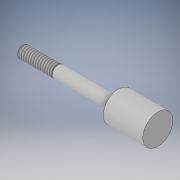
# Autodesk Inventor part: 0070.0110000_rod
Saved by Autodesk Inventor 2018 (Build 220112000, 112)
## iProperties
Created: 2019-01-16
Part Number: 0070.0110000_rod
Material: Generic
Catalog Web Link: www.cadenas.de
Description: Standard Air Cylinder_rod-Original Line - Standard Air Cylinders
Vendor: BIMBA
Document SubType Name: Modeling
Designer: s-4008082
Manufacturer: BIMBA
Mass: 0.744089 g
Surface Area: 6.29772 cm^2
Volume: 0.744089 cm^3
Density: 1 g/cm^3
Appearance: PSOLRGB-181-181-181
Category: PARTsolutions
Company: BIMBA
Title: 0070.0110000_rod
Author: Cadenas PARTsolutions
Comments: Original Line - Standard Air Cylinders
PSOL_IDENT_0: {$CADENAS_DATA\23d-libs\bimba\bimba\bimba_imperial\bimba_full_line\original_line_cylinders\standard_
PSOL_IDENT_1: air_cylinders\rod.prj},325 {VTYP=3D},{NB=0070.0110000_rod},{LINA=0070.0110000_rod},{NN=Standard Air
PSOL_IDENT_2: Cylinder_rod},{DATE=21.03.2018 14:31:21},{GEOMDATE=09.11.2017 13:09:15},{VERSION=},{LINEID=20},{WBVA
PSOL_IDENT_3: R=STROKE,ACTING,MNT,DER,NR,BM,CO,M,EE,EEL,K,Q,Y,F,G,T,B,H,SER,SR,NT,W,E,HL,ST,STP,PRC,PB,COLOR1,FCD,
PSOL_IDENT_4: RCD,BCD},{WBNUMERIC=STROKE,EEL,COLOR1,FCD,RCD,BCD}  {NB=0070.0110000_rod},{LINA=0070.0110000_rod},{K
PSOL_IDENT_5: T=DUMMY},{PN=0070.011000},{DASH=},{BORE=0.31250000},{BOREPN=007},{STROKE=0.011},{STROKEALG=[0.001:50
PSOL_IDENT_6: /0.001]},{STROKE1=0.011},{ACTING=},{ACTINGALG= '' , 'Single Acting' , 'R' , 'Reverse Single Acting'
PSOL_IDENT_7: , 'D' , 'Double Acting' },{ACTINGPN=},{MNT=},{MNTALG= '' , 'Front Nose Mounting' , 'XP' , 'Double En
PSOL_IDENT_8: d or Rear Pivot Mounting' },{TYPE=},{MNTPN=},{DER=},{DERALG= '' , 'N/A' },{NR=},{NRALG= '' , 'N/A' }
PSOL_IDENT_9: ,{NRPN=},{BM=},{BMALG= '' , 'N/A' },{BMPN=},{CO=},{COALG= '' , 'N/A' },{M=},{MALG= '', 'Without Magn
PSOL_IDENT_10: et', 'M', 'With Magnet' },{EE=},{EEL=0},{EEMAX=50},{EEALG= '', 'Without Extra Extension', 'EE', 'Wit
PSOL_IDENT_11: h Extra Extension' },{EELALG=0},{EEPN=},{EEPN1=0.000},{K=},{KALG= '' , 'N/A' },{KPN=},{Q=},{QALG= ''
PSOL_IDENT_12: , 'Without Side Ported Rear Head' , 'Q' , 'With Side Ported Rear Head' },{QPN=},{Y=},{YALG= '' , 'N
PSOL_IDENT_13: /A' },{YPN=},{F=},{FALG= '', 'Standard', 'F', 'Molycoated Body' },{FPN=},{G=},{GPN=},{T=},{TALG= ''
PSOL_IDENT_14: , 'Standard' , 'N' , 'Low Temperature' , 'V' , 'High Temperature' },{NPN=},{VPN=},{B=},{BALG= '' , '
PSOL_IDENT_15: With Bumper' },{BPN=},{H=},{HALG= '', 'N/A' },{HPN=},{SER=},{SERALG= '' , 'N/A' },{SR=},{SRALG= 'C'
PSOL_IDENT_16: , 'Carbon Steel Rod' , 'SR' , '303 Stainless Steel Rod' , '' , '303 Stainless Steel Rod1' },{SRPN=},
PSOL_IDENT_17: {SRCON=0},{NT=},{NTPN=},{W=},{WALG= '' , 'N/A' },{WPN=},{E=},{EALG= '' , 'Without Special Lube and S
PSOL_IDENT_18: eals' , 'E' , 'With Special Lube and Seals' },{EPN=},{HL=},{HLALG= '' , 'N/A' },{ST=},{STALG= '' , '
PSOL_IDENT_19: Without Switch Track' , 'T' , 'With Switch Track' },{STP=},{STPALG= '' , 'N/A' },{STPN=},{PRC=},{PRC
PSOL_IDENT_20: ALG= '' , 'Without Piston Rod Clevis' , 'D-166-1' , 'With Piston Rod Clevis' },{PRCPN=},{PB=},{PBALG=
PSOL_IDENT_21: '' , 'Without Pivot Bracket' , 'D-167' , 'With Pivot Bracket' },{PBPN=},{TLEN=0.7975},{TEXT=0.10073
PSOL_IDENT_22: 3},{SPACE=0.057562},{FRAC=1.3810},{RGCON=},{RGDACCON=},{RHCON=},{RHCONON=1},{RHACCON=},{FNUTCON=1},{
PSOL_IDENT_23: RNUTCON=0},{FNUTPN=D-344},{RNUTPN=},{FNUTTRANS=0.0000},{RNUTTRANS=0.0000},{VHOLECON=2},{A1=0.6250},{
PSOL_IDENT_24: A1N=0.6250},{A1P=0.8450},{A1B=0.9060},{A4=0.2550},{A4N=0.2550},{A4P=0.1585},{A5=0.0220},{A1H=0.328},
PSOL_IDENT_25: {A1NH=0.3280},{A1PH=0.8750},{A1BH=0.0000},{A1SH=0.0000},{A2H=0.1585},{A2NH=0.1585},{LENGTH=1.1200},{
PSOL_IDENT_26: LENGTH1=1.1200},{LENGTH2=1.6500},{MUL=0.0083},{MUL11=0.0083},{MUL22=0.0137},{MUL33=0.0083},{MUL2=0.7
PSOL_IDENT_27: 500},{MUL211=0.7500},{MUL222=1.2500},{MUL233=0.7500},{SSS=0.0110},{RGLEN=0.3920},{RHLEN=0.1915},{SSS
PSOL_IDENT_28: 1=1.0000},{A13=0.7190},{THDLEN1=0.3800},{THD1=0.1250},{TAB=UNC},{THDLEN=0.3800},{THD=0.1250},{OD=0.3
PSOL_IDENT_29: 215},{RODL=1.4330},{PL=0.4170},{RODDIA=0.1250},{HEX=0.0000},{RODTRANS=0.0000},{G1=0.0000},{ON=0},{G5=
PSOL_IDENT_30: 0.0000},{DERLEN=1.0160},{THOLE=0.0000},{WF=0.0000},{BADD=0.0000},{MADD=0.0000},{NVADD=0.000},{JRADD=
PSOL_IDENT_31: 0.00000},{COLOR=0.71,0.71,0.71,0.00},{GROOVE=1},{HOL=0},{D7=0.1270},{H1=0.0000},{D1=0.3590},{D1RH=0.
PSOL_IDENT_32: 3590},{D1P=0.0000},{D1B=0.6050},{D1N=0.3590},{D1NRH=0.3590},{D1BRH=0.0000},{D1PRH=0.4380},{BOZO=0},{
PSOL_IDENT_33: HADD=0.000},{COLOR1=0},{DEFL=0.0000},{HEXL=0.0000},{SSADD=0.0000},{WFL=0.0000},{MOVE=0.0000},{PRCL2=
PSOL_IDENT_34: 0.18800},{PRCB=0.11000},{PRCTRANS=0.00000},{FCD=0},{RCD=0},{BCD=0}
NN: Standard Air Cylinder_rod
NT: Standard
NB: 0070.0110000_rod
NBSYN: $PN.$COLOR1._rod
LINA: 0070.0110000_rod
PN: 0070.011000
BORE: 0.3125
BOREPN: 007
STROKE: 0.011
ACTING: Single Acting
MNT: Front Nose Mounting
DER: N/A
NR: N/A
BM: N/A
CO: N/A
M: Without Magnet
EE: Without Extra Extension
EEL: 0
K: N/A
Q: Without Side Ported Rear Head
Y: N/A
F: Standard
G: Without Magnalube Lubrication
T: Standard
B: With Bumper
H: N/A
SER: N/A
SR: 303 Stainless Steel Rod1
W: N/A
E: Without Special Lube and Seals
HL: N/A
ST: Without Switch Track
STP: N/A
PRC: Without Piston Rod Clevis
PB: Without Pivot Bracket
A1N: 0.625
A1P: 0.845
A1B: 0.906
A4N: 0.255
A4P: 0.1585
A5: 0.022
A1NH: 0.328
A1PH: 0.875
A1BH: 0
A1SH: 0
A2NH: 0.1585
A13: 0.719
THDLEN1: 0.38
THD1: 0.125
TAB: UNC
OD: 0.3215
RODDIA: 0.125
HEX: 0
G1: 0
G5: 0
THOLE: 0
WF: 0
GROOVE: 1
D7: 0.127
D1P: 0
D1B: 0.605
D1N: 0.359
D1NRH: 0.359
D1BRH: 0
D1PRH: 0.438
COLOR1: 0
FCD: 0
RCD: 0
BCD: 0
SUPPLIER: BIMBA
ARTICLENO: 0070.0110000_rod
BOMINFO: 0070.0110000_rod
CREATOR: CADENAS GmbH
Autodesk Inventor part; units mm, degrees
sketch "Sketch_1" plane through (0, 0, 0) normal (0, 0, 1) x (1, 0, 0)
  line L0 (26.7462, 0) -> (0, 0)
  line L1 (0, 0) -> (0, 1.5875)
  line L2 (0, 1.5875) -> (16.1544, 1.5875)
  line L3 (16.1544, 1.5875) -> (16.1544, 4.0323)
  line L4 (16.1544, 4.0323) -> (26.7462, 4.0323)
  line L5 (26.7462, 4.0323) -> (26.7462, 0)
  line L6 (26.7462, 0) -> (0, 0)
  constraints: 14 end point
revolve "Revolution1" add sketch "Sketch_1" angle 360 about axis through (26.7462, 0, 0) along (1, 0, 0)
sketch "Sketch_2" plane through (0, 0, 0) normal (0, 0, 1) x (1, 0, 0)
  line L0 (0, 0) -> (-9.652, 0)
  line L1 (-9.652, 0) -> (-9.652, 1.209)
  line L2 (-9.652, 1.209) -> (-9.2735, 1.5875)
  line L3 (-9.2735, 1.5875) -> (0, 1.5875)
  line L4 (0, 1.5875) -> (0, 0)
  line L5 (0, 0) -> (-9.652, 0)
  constraints: 12 end point
revolve "Revolution2" add sketch "Sketch_2" angle 360 about axis through (0, 0, 0) along (1, 0, 0)
thread "Thread1" size "5-40 UNC" class "2A" standard "ANSI Unified Screw Threads" length 9.2735
sketch "Sketch_30" plane through (0, 0, 0) normal (0, 0, 1) x (1, 0, 0)
  line L0 (0, 0) -> (-0.254, 0)
  line L1 (-0.254, 1.3335) -> (0, 1.3335)
  line L2 (0, 1.3335) -> (0, 1.8415)
  line L3 (0, 1.8415) -> (-0.254, 1.8415)
  line L4 (-0.254, 1.8415) -> (-0.254, 1.3335)
  constraints: 10 end point
revolve "Revolution3" cut sketch "Sketch_30" angle 360 about axis through (0, 0, 0) along (1, 0, 0)
ref_plane "dia1_XY" through (0, 1.5875, 0) normal (1, 0, 0) x (0, 0, -1)
ref_plane "dia1_YZ" through (0, 1.5875, 0) normal (0, 0, -1) x (0, 1, 0)
ref_plane "dia1_ZX" through (0, 1.5875, 0) normal (0, 1, 0) x (1, 0, 0)
ref_plane "dia12_XY" through (0, 0, 4.5593) normal (1, 0, 0) x (0, 0, -1)
ref_plane "dia12_YZ" through (0, 0, 4.5593) normal (0, 0, -1) x (0, 1, 0)
ref_plane "dia12_ZX" through (0, 0, 4.5593) normal (0, 1, 0) x (1, 0, 0)
ref_plane "dia2_XY" through (0, -1.5875, 0) normal (1, 0, 0) x (0, 0, -1)
ref_plane "dia2_YZ" through (0, -1.5875, 0) normal (0, 0, -1) x (0, 1, 0)
ref_plane "dia2_ZX" through (0, -1.5875, 0) normal (0, 1, 0) x (1, 0, 0)
ref_plane "dia22_XY" through (0, 0, -4.5593) normal (1, 0, 0) x (0, 0, -1)
ref_plane "dia22_YZ" through (0, 0, -4.5593) normal (0, 0, -1) x (0, 1, 0)
ref_plane "dia22_ZX" through (0, 0, -4.5593) normal (0, 1, 0) x (1, 0, 0)
ref_plane "rl1_XY" through (-9.652, 0, 0) normal (1, 0, 0) x (0, 0, -1)
ref_plane "rl1_YZ" through (-9.652, 0, 0) normal (0, 0, -1) x (0, 1, 0)
ref_plane "rl1_ZX" through (-9.652, 0, 0) normal (0, 1, 0) x (1, 0, 0)
ref_plane "rl2_XY" through (0, 0, 0) normal (1, 0, 0) x (0, 0, -1)
ref_plane "rl2_YZ" through (0, 0, 0) normal (0, 0, -1) x (0, 1, 0)
ref_plane "rl2_ZX" through (0, 0, 0) normal (0, 1, 0) x (1, 0, 0)
ref_plane "rod_cp_XY" through (0, 0, 0) normal (1, 0, 0) x (0, 0, -1)
ref_plane "rod_cp_YZ" through (0, 0, 0) normal (0, 0, -1) x (0, 1, 0)
ref_plane "rod_cp_ZX" through (0, 0, 0) normal (0, 1, 0) x (1, 0, 0)
ref_plane "thd1_XY" through (-9.652, 1.5875, 0) normal (1, 0, 0) x (0, 0, -1)
ref_plane "thd1_YZ" through (-9.652, 1.5875, 0) normal (0, 0, -1) x (0, 1, 0)
ref_plane "thd1_ZX" through (-9.652, 1.5875, 0) normal (0, 1, 0) x (1, 0, 0)
ref_plane "thd2_XY" through (-9.652, -1.5875, 0) normal (1, 0, 0) x (0, 0, -1)
ref_plane "thd2_YZ" through (-9.652, -1.5875, 0) normal (0, 0, -1) x (0, 1, 0)
ref_plane "thd2_ZX" through (-9.652, -1.5875, 0) normal (0, 1, 0) x (1, 0, 0)
ref_plane "to_rod_clevis_XY" through (-9.652, 0, 0) normal (1, 0, 0) x (0, 0, -1)
ref_plane "to_rod_clevis_YZ" through (-9.652, 0, 0) normal (0, 0, -1) x (0, 1, 0)
ref_plane "to_rod_clevis_ZX" through (-9.652, 0, 0) normal (0, 1, 0) x (1, 0, 0)
body "Solid1"
